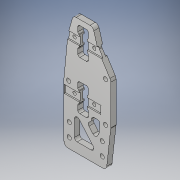
# Autodesk Inventor part: 前後機構_上側板
Saved by Autodesk Inventor 2019.4 (Build 234330000, 330)
## iProperties
Created: 2021-12-05
Part Number: 前後機構_上側板
Material: アルミニウム 6061
Document SubType Name: Modeling
Designer: 堀川皓史
Density: 2.7 g/cm^3
Appearance: アルミニウム - フラット
Author: 堀川皓史
Autodesk Inventor part; units mm, degrees
ref_plane "YZ Plane" through (0, 0, 0) normal (1, 0, 0) x (0, 1, 0)
ref_plane "XZ Plane" through (0, 0, 0) normal (0, 1, 0) x (-1, 0, 0)
ref_plane "XY Plane" through (0, 0, 0) normal (0, 0, 1) x (1, 0, 0)
sketch "スケッチ1" plane through (0, 0, 0) normal (0, 0, 1) x (1, 0, 0)
  line L0 (-7.5, 51.6667) -> (7.5, 51.6667) construction
  line L1 (7.5, 51.6667) -> (7.5, -56.5972) construction
  line L2 (7.5, -56.5972) -> (-7.5, -56.5972) construction
  line L3 (-7.5, -56.5972) -> (-7.5, 51.6667) construction
  circle A0 centre (-11, 0) radius 3.5 construction
  circle A1 centre (17, 15) radius 9.5 construction
  circle A2 centre (17, -15) radius 9.5 construction
  circle A3 centre (-11, 0) radius 1.6
  line L4 (17, 15) -> (17, -15) construction
  line L5 (17, -15) -> (-11, 0) construction
  line L6 (-11, 0) -> (17, 15) construction
  circle A4 centre (17, 15) radius 1.6
  circle A5 centre (17, -15) radius 1.6
  line L7 (-3.1, 34) -> (-3.1, 26)
  arc A6 (3.1, 26) -> (3.325, 25.5824) centre (3.6, 26) ccw
  line L8 (3.1, 34) -> (3.1, 26)
  arc A7 (4, 24.3297) -> (3.325, 25.5824) centre (2.5, 24.3297) ccw
  line L9 (4, 21) -> (4, 24.3297)
  line L10 (-3, 20.5) -> (-3, 39.5) construction
  line L11 (3, 39.5) -> (3, 20.5) construction
  arc A8 (-3.325, 25.5824) -> (-4, 24.3297) centre (-2.5, 24.3297) ccw
  arc A9 (-3.325, 25.5824) -> (-3.1, 26) centre (-3.6, 26) ccw
  arc A10 (-4, 21) -> (-2.5, 19.5) centre (-2.5, 21) ccw
  line L12 (-4, 24.3297) -> (-4, 21)
  arc A11 (4, 39) -> (2.5, 40.5) centre (2.5, 39) ccw
  line L13 (-2.5, 19.5) -> (2.5, 19.5)
  line L14 (3, 20.5) -> (-3, 20.5) construction
  arc A12 (2.5, 19.5) -> (4, 21) centre (2.5, 21) ccw
  arc A13 (3.325, 34.4176) -> (3.1, 34) centre (3.6, 34) ccw
  arc A14 (3.325, 34.4176) -> (4, 35.6703) centre (2.5, 35.6703) ccw
  arc A15 (-3.1, 34) -> (-3.325, 34.4176) centre (-3.6, 34) ccw
  arc A16 (-4, 35.6703) -> (-3.325, 34.4176) centre (-2.5, 35.6703) ccw
  line L15 (4, 35.6703) -> (4, 39)
  line L16 (-4, 39) -> (-4, 35.6703)
  line L17 (-3, 39.5) -> (3, 39.5) construction
  line L18 (2.5, 40.5) -> (-2.5, 40.5)
  arc A17 (-2.5, 40.5) -> (-4, 39) centre (-2.5, 39) ccw
  line L19 (-3.1, -3) -> (-3.1, -11)
  arc A18 (3.1, -11) -> (3.325, -11.4176) centre (3.6, -11) ccw
  line L20 (3.1, -3) -> (3.1, -11)
  arc A19 (4, -12.6703) -> (3.325, -11.4176) centre (2.5, -12.6703) ccw
  line L21 (4, -16) -> (4, -12.6703)
  line L22 (-3, -16.5) -> (-3, 2.5) construction
  line L23 (3, 2.5) -> (3, -16.5) construction
  arc A20 (-3.325, -11.4176) -> (-4, -12.6703) centre (-2.5, -12.6703) ccw
  arc A21 (-3.325, -11.4176) -> (-3.1, -11) centre (-3.6, -11) ccw
  arc A22 (-4, -16) -> (-2.5, -17.5) centre (-2.5, -16) ccw
  line L24 (-4, -12.6703) -> (-4, -16)
  arc A23 (4, 2) -> (2.5, 3.5) centre (2.5, 2) ccw
  line L25 (-2.5, -17.5) -> (2.5, -17.5)
  line L26 (3, -16.5) -> (-3, -16.5) construction
  arc A24 (2.5, -17.5) -> (4, -16) centre (2.5, -16) ccw
  arc A25 (3.325, -2.5824) -> (3.1, -3) centre (3.6, -3) ccw
  arc A26 (3.325, -2.5824) -> (4, -1.3297) centre (2.5, -1.3297) ccw
  arc A27 (-3.1, -3) -> (-3.325, -2.5824) centre (-3.6, -3) ccw
  arc A28 (-4, -1.3297) -> (-3.325, -2.5824) centre (-2.5, -1.3297) ccw
  line L27 (4, -1.3297) -> (4, 2)
  line L28 (-4, 2) -> (-4, -1.3297)
  line L29 (-3, 2.5) -> (3, 2.5) construction
  line L30 (2.5, 3.5) -> (-2.5, 3.5)
  arc A29 (-2.5, 3.5) -> (-4, 2) centre (-2.5, 2) ccw
  circle A30 centre (-7.5, 30) radius 1.25
  circle A31 centre (7.5, 30) radius 1.25
  circle A32 centre (-7.5, -7) radius 1.25
  circle A33 centre (7.5, -7) radius 1.25
  arc A34 (-14.4827, 0.348) -> (-14.5, 0) centre (-11, 0) ccw
  line L31 (-7.5, 44.5) -> (7.5, 44.5)
  arc A35 (21, 15) -> (20.3793, 17.1402) centre (17, 15) ccw
  arc A36 (20.9744, -15.4516) -> (21, -15) centre (17, -15) ccw
  line L32 (-14.5, -44.5) -> (17.6735, -44.5)
  circle A37 centre (-10.5, -37) radius 1.6
  circle A38 centre (14.5, -27) radius 1.6
  circle A39 centre (14.5, -37) radius 1.6
  line L33 (-14.5, -19.5) -> (33.1902, -19.5) construction
  line L34 (33.1902, -19.5) -> (33.1902, -44.5) construction
  line L35 (33.1902, -44.5) -> (-14.5, -44.5) construction
  line L36 (-14.5, -44.5) -> (-14.5, -19.5) construction
  arc A40 (-11.3448, 31.1034) -> (-11.4802, 30.3977) centre (-7.5, 30) ccw
  line L37 (-7.5, 44.5) -> (-11.3448, 31.1034)
  line L38 (-11.4802, 30.3977) -> (-14.4827, 0.348)
  line L39 (7.5, 44.5) -> (11.1864, 31.6552)
  line L40 (11.1864, 31.6552) -> (20.3793, 17.1402)
  arc A41 (11.4653, 29.4746) -> (11.0874, 31.7692) centre (7.5, 30) ccw construction
  line L41 (21, 15) -> (21, -15)
  circle A42 centre (-10.5, -27) radius 1.6
  line L42 (-14.5, 0) -> (-14.5, -44.5)
  line L43 (20.9744, -15.4516) -> (17.6735, -44.5)
  point P0 (0, 0)
  point P1 (0, 0)
  point P2 (0, 30)
  point P3 (0, -7)
  dimension "d0" = 15
  dimension "d1" = 7.5
  dimension "d2" = 7
  dimension "d3" = 19
  dimension "d4" = 19
  dimension "d5" = 3.2
  dimension "d10" = 30
  dimension "d11" = 3.2
  dimension "d12" = 3.2
  dimension "d13" = 6
  dimension "d14" = 19
  dimension "d15" = 3
  dimension "d16" = 9.5
  dimension "d17" = 1
  dimension "d18" = 8
  dimension "d19" = 4
  dimension "d20" = 0.1
  dimension "d21" = 0.1
  dimension "d22" = 1
  dimension "d23" = 1
  dimension "d24" = 1
  dimension "d25" = 1.5
  dimension "d26" = 1
  dimension "d27" = 1.5
  dimension "d28" = 0.5
  dimension "d29" = 1
  dimension "d30" = 1.5
  dimension "d31" = 0.5
  dimension "d32" = 1.5
  dimension "d33" = 0.5
  dimension "d34" = 0.5
  dimension "d35" = 1.5
  dimension "d36" = 6
  dimension "d37" = 19
  dimension "d38" = 3
  dimension "d39" = 9.5
  dimension "d40" = 1
  dimension "d41" = 8
  dimension "d42" = 4
  dimension "d43" = 0.1
  dimension "d44" = 0.1
  dimension "d45" = 1
  dimension "d46" = 1
  dimension "d47" = 1
  dimension "d48" = 1.5
  dimension "d49" = 1
  dimension "d50" = 1.5
  dimension "d51" = 0.5
  dimension "d52" = 1
  dimension "d53" = 1.5
  dimension "d54" = 0.5
  dimension "d55" = 1.5
  dimension "d56" = 0.5
  dimension "d57" = 0.5
  dimension "d58" = 1.5
  dimension "d59" = 30
  dimension "d60" = 7
  dimension "d61" = 2.5
  dimension "d62" = 2.5
  dimension "d63" = 2.5
  dimension "d64" = 2.5
  dimension "d65" = 15
  dimension "d66" = 7.5
  dimension "d68" = 15
  constraints: 88 end point, 58 point on circle, 50 tangent, 43 centre point, 15 horizontal alignment, 14 parallel, 8 coincident, 8 perpendicular, 8 vertical, 6 equal radius, 5 vertical alignment, 4 horizontal, 2 point on line, 1 equal length
  measures "d0" distance between parallel lines of L1 L3
  measures "d1" distance from line of point (0, 0) L3
  measures "d2" diameter of A0
  measures "d3" diameter of A1
  measures "d4" diameter of A2
  measures "d5" diameter of A3
  measures "d10" distance of L4.start L4.end
  measures "d11" diameter of A4
  measures "d12" diameter of A5
  measures "d13" distance of L17.start L17.end
  measures "d14" distance of L17.end L14.start
  measures "d15" distance from line of point (0, 30) L10
  measures "d16" distance from line of point (0, 30) L17
  measures "d17" distance between parallel lines of L14 L13
  measures "d18" distance of L7.start L7.end
  measures "d19" vertical distance of point (0, 30) L7.end
  measures "d20" distance between parallel lines of L7 L10
  measures "d21" distance between parallel lines of L11 L8
  measures "d22" distance between parallel lines of L10 L12
  measures "d23" distance between parallel lines of L11 L9
  measures "d24" distance between parallel lines of L17 L18
  measures "d25" radius of A17
  measures "d26" distance between parallel lines of L10 L16
  measures "d27" radius of A16
  measures "d28" radius of A15
  measures "d29" distance between parallel lines of L11 L15
  measures "d30" radius of A14
  measures "d31" radius of A13
  measures "d32" radius of A8
  measures "d33" radius of A9
  measures "d34" radius of A6
  measures "d35" radius of A7
  measures "d36" distance of L29.start L29.end
  measures "d37" distance of L29.end L26.start
  measures "d38" distance from line of point (0, -7) L22
  measures "d39" distance from line of point (0, -7) L29
  measures "d40" distance between parallel lines of L26 L25
  measures "d41" distance of L19.start L19.end
  measures "d42" vertical distance of point (0, -7) L19.end
  measures "d43" distance between parallel lines of L19 L22
  measures "d44" distance between parallel lines of L23 L20
  measures "d45" distance between parallel lines of L22 L24
  measures "d46" distance between parallel lines of L23 L21
  measures "d47" distance between parallel lines of L29 L30
  measures "d48" radius of A29
  measures "d49" distance between parallel lines of L22 L28
  measures "d50" radius of A28
  measures "d51" radius of A27
  measures "d52" distance between parallel lines of L23 L27
  measures "d53" radius of A26
  measures "d54" radius of A25
  measures "d55" radius of A20
  measures "d56" radius of A21
  measures "d57" radius of A18
  measures "d58" radius of A19
  measures "d59" distance of point (0, 0) point (0, 30)
  measures "d60" distance of point (0, 0) point (0, -7)
  measures "d61" diameter of A30
  measures "d62" diameter of A31
  measures "d63" diameter of A32
  measures "d64" diameter of A33
  measures "d65" distance of A31.centre A30.centre
  measures "d66" distance of point (0, 30) A30.centre
  measures "d68" distance of A33.centre A32.centre
extrude "押し出し1" add sketch "スケッチ1" along normal blind 4
sketch "スケッチ2" plane through (0, 0, 4) normal (0, 0, 1) x (1, 0, 0)
  line L0 (-13, 33) -> (17, 33)
  line L1 (17, 33) -> (17, 27)
  line L2 (17, 27) -> (-13, 27)
  line L3 (-13, 27) -> (-13, 33)
  line L4 (-14.4, -4) -> (13.6, -4)
  line L5 (13.6, -4) -> (13.6, -10)
  line L6 (13.6, -10) -> (-14.4, -10)
  line L7 (-14.4, -10) -> (-14.4, -4)
  circle A0 centre (-7.5, 30) radius 1.25 projected
  circle A1 centre (-7.5, -7) radius 1.25 projected
  point P0 (0, 0)
  dimension "d97" = 6
  dimension "d98" = 3
  dimension "d99" = 3
  dimension "d100" = 6
  dimension "d103" = 28
  dimension "d104" = 6.9
  dimension "d105" = 30
  dimension "d106" = 5.5
  constraints: 16 end point, 4 parallel, 2 horizontal, 2 perpendicular
  measures "d97" distance between parallel lines of L2 L0
  measures "d98" distance from line of L0 A0.centre
  measures "d99" distance from line of A1.centre L4
  measures "d100" distance of L6.end L4.start
  measures "d103" distance of L5.end L6.end
  measures "d104" distance from line of A1.centre L7
  measures "d105" distance of L1.end L2.end
  measures "d106" distance from line of A0.centre L3
extrude "押し出し2" cut sketch "スケッチ2" against normal blind 1
sketch "スケッチ3" plane through (0, 0, 4) normal (0, 0, 1) x (1, 0, 0)
  line L0 (-6.5, -37) -> (10.5, -37)
  line L1 (10.5, -37) -> (-6.5, -17.1901)
  line L2 (-6.5, -17.1901) -> (-6.5, -37)
  line L3 (2.5, -17.5) -> (-2.5, -17.5) construction
  line L4 (-14.5, -44.5) -> (17.6735, -44.5) projected
  line L5 (-14.5, 0) -> (-14.5, -44.5) projected
  circle A0 centre (-10.5, -37) radius 1.6 construction
  circle A1 centre (14.5, -37) radius 1.6 construction
  line L6 (17.6735, -44.5) -> (20.9744, -15.4516) projected
  circle A2 centre (17, -15) radius 1.6 construction
  circle A3 centre (14.5, -27) radius 1.6 construction
  arc A4 (11.962, -23.9083) -> (10.5, -27) centre (14.5, -27) ccw
  line L7 (13.0256, -14.5484) -> (11.962, -23.9083)
  circle A5 centre (17, -15) radius 4 construction
  circle A6 centre (-10.5, -37) radius 4 construction
  circle A7 centre (14.5, -37) radius 4 construction
  line L8 (10.5, -27) -> (10.5, -29.3223)
  line L9 (10.5, -29.3223) -> (2.5, -20)
  line L10 (13.0256, -14.5484) -> (6.5, -14.5484)
  arc A8 (2.5, -20) -> (6.5, -16) centre (2.5, -16) ccw
  line L11 (14.5, -27) -> (14.5, -37) construction
  arc A9 (2.5, -17.5) -> (4, -16) centre (2.5, -16) ccw construction
  line L12 (6.5, -16) -> (6.5, -14.5484)
  line L13 (6.5, -14.5484) -> (6.2273, -14.5484) construction
  arc A10 (6.5, -16) -> (6.2273, -14.5484) centre (2.5, -16) ccw construction
  point P0 (0, 0)
  dimension "d117" = 8
  dimension "d118" = 8
  dimension "d119" = 8
  dimension "d114" = 4
  dimension "d116" = 8
  dimension "d120" = 4
  dimension "d121" = 5
  dimension "d122" = 4
  constraints: 20 end point, 8 point on circle, 5 coincident, 3 centre point, 3 horizontal, 3 parallel, 3 vertical, 2 horizontal alignment, 2 perpendicular, 1 point on line, 1 tangent, 1 vertical alignment, 7 other
  measures "d114" radius of A4
  measures "d116" distance between parallel lines of L6 L7
  measures "d120" distance between parallel lines of L11 L8
  measures "d121" distance between parallel lines of L1 L9
  measures "d122" radius of A8
extrude "押し出し3" cut sketch "スケッチ3" against normal through all
fillet "フィレット1" radius 2 8 edges at (6.5, -14.5484, 2) (13.0256, -14.5484, 2) (11.962, -23.9083, 2) (2.5, -20, 2) (10.5, -29.3223, 2) (-6.5, -17.1901, 2) (-6.5, -37, 2) (10.5, -37, 2)
fillet "フィレット2" radius 3 5 edges at (-7.5, 44.5, 2) (7.5, 44.5, 2) (11.1864, 31.6552, 1.5) (17.6735, -44.5, 2) (-14.5, -44.5, 2)
sketch "スケッチ4" plane through (0, 0, 0) normal (0, 0, -1) x (-1, 0, 0)
  line L0 (-16.5372, 33) -> (16.1705, 33)
  line L1 (16.1705, 33) -> (16.1705, 27)
  line L2 (16.1705, 27) -> (-16.5372, 27)
  line L3 (-16.5372, 27) -> (-16.5372, 33)
  line L4 (-13.6, -4) -> (14.4, -4)
  line L5 (14.4, -4) -> (14.4, -10)
  line L6 (14.4, -10) -> (-13.6, -10)
  line L7 (-13.6, -10) -> (-13.6, -4)
  circle A0 centre (7.5, 30) radius 1.25 projected
  circle A1 centre (7.5, -7) radius 1.25 projected
  point P0 (0, 0)
  dimension "d127" = 3
  dimension "d128" = 6
  dimension "d129" = 3
  dimension "d130" = 6
  dimension "d131" = 28
  dimension "d132" = 6.9
  constraints: 16 end point, 4 parallel, 2 horizontal, 2 perpendicular
  measures "d127" distance from line of L0 A0.centre
  measures "d128" distance of L0.end L1.end
  measures "d129" distance from line of A1.centre L4
  measures "d130" distance of L4.end L5.end
  measures "d131" distance of L5.end L6.end
  measures "d132" distance from line of A1.centre L5
extrude "押し出し4" cut sketch "スケッチ4" against normal blind 1
equation "\"d1\" = 0.5 * d0"
equation "\"d16\" = 0.5 * d14"
equation "\"d39\" = 0.5 * d37"
